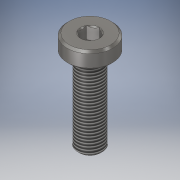
# Autodesk Inventor part: Bolt_M3x0.35_10mm_LSH
Saved by Autodesk Inventor 2018 (Build 220112000, 112)
## iProperties
Manager: Bradley
Created: 2016-07-03
Part Number: Bolt_M3x0.35_10mm_LSH
Material: Stainless Steel
Document SubType Name: Modeling
Designer: Bradley
Density: 8 g/cm^3
Appearance: Semi-Polished
Author: Bradley
Autodesk Inventor part; units mm, degrees
ref_plane "YZ Plane" through (0, 0, 0) normal (1, 0, 0) x (0, 1, 0)
ref_plane "XZ Plane" through (0, 0, 0) normal (0, 1, 0) x (-1, 0, 0)
ref_plane "XY Plane" through (0, 0, 0) normal (0, 0, 1) x (1, 0, 0)
sketch "Sketch1" plane through (0, 0, 0) normal (0, 0, 1) x (1, 0, 0)
  line L0 (0, 6) -> (0, -6)
  line L1 (0, -6) -> (1.25, -6)
  line L2 (1.25, -6) -> (1.5, -5.75)
  line L3 (1.5, -5.75) -> (1.5, 3.9)
  line L4 (1.6, 4) -> (2.5, 4)
  line L5 (2.75, 4.25) -> (2.75, 5.75)
  line L6 (2.5, 6) -> (0, 6)
  arc A0 (1.6, 4) -> (1.5, 3.9) centre (1.6, 3.9) ccw
  line L7 (2.5, 6) -> (2.75, 5.75)
  line L8 (2.5, 4) -> (2.75, 4.25)
  point P0 (0, 0)
  point P1 (2.75, 4)
  point P2 (2.75, 6)
  point P3 (0, 0)
  dimension "d0" = 5.5
  dimension "d1" = 2
  dimension "d3" = 3
  dimension "d4" = 3.2
  dimension "d5" = 135
  dimension "d6" = 0.25
  dimension "d7" = 10
  dimension "d9" = 0.25
  constraints: 18 end point, 6 perpendicular, 4 point on line, 2 point on circle, 2 tangent, 1 centre point, 1 coincident, 1 midpoint, 1 parallel, 1 vertical, 1 vertical alignment
  measures "d0" diameter of L5 L0
  measures "d1" distance of point (2.75, 4) point (2.75, 6)
  measures "d3" diameter of L3 L0
  measures "d4" diameter of L4.start L0
  measures "d5" angle of L3 L2
  measures "d6" horizontal distance of L1.end L2.end
  measures "d7" distance between parallel lines of L1 L4
  measures "d9" distance of L6.start point (2.75, 6)
revolve "Revolution1" add sketch "Sketch1" angle 360 about axis through (0, 6, 0) along (0, -1, 0)
sketch "Sketch2" plane through (0, 6, 0) normal (0, 1, 0) x (1, 0, 0)
  line L0 (0, -1.1547) -> (-1, -0.5774)
  line L1 (-1, -0.5774) -> (-1, 0.5774)
  line L2 (-1, 0.5774) -> (0, 1.1547)
  line L3 (0, 1.1547) -> (1, 0.5774)
  line L4 (1, 0.5774) -> (1, -0.5774)
  line L5 (1, -0.5774) -> (0, -1.1547)
  point P0 (0, 0)
  point P1 (0, 0)
  dimension "d11" = 2
  constraints: 12 end point, 1 coincident, 1 vertical, 13 other
  measures "d11" distance between parallel lines of L4 L1
extrude "Extrusion1" cut sketch "Sketch2" against normal blind 1.5
thread "Thread1" size "M3x0.35" class "6g" standard "ANSI Metric M Profile" full length
sketch "Sketch3" plane through (0, 0, 0) normal (1, 0, 0) x (0, 1, 0)
  line L0 (6, 1.1547) -> (5, 0.1547)
  line L1 (5, 0.1547) -> (6, 0.1547)
  line L2 (6, 0.1547) -> (6, 1.1547)
  line L3 (-1.4, 0) -> (8.4, 0) projected
  point P0 (0, 0)
  dimension "d18" = 1
  constraints: 6 end point, 2 perpendicular, 1 vertical
  measures "d18" distance of L1.end L0.start
revolve "Revolution2" cut sketch "Sketch3" angle 360 about axis through (0, -10, 0) along (0, 1, 0)
body "Solid1"
